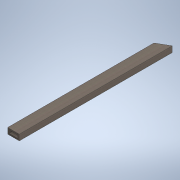
# Autodesk Inventor part: 1x0_5x12-aluminumExtrusion
Saved by Autodesk Inventor 2020.2 (Build 242310000, 310)
## iProperties
Created: 2020-01-20
Part Number: 1x0_5x12-aluminumExtrusion
Material: Aluminum 6061, Welded
Document SubType Name: Modeling
Designer: robst
Density: 2.7 g/cm^3
Appearance: Walnut
Author: robst
Autodesk Inventor part; units mm, degrees
ref_plane "YZ Plane" through (0, 0, 0) normal (1, 0, 0) x (0, 1, 0)
ref_plane "XZ Plane" through (0, 0, 0) normal (0, 1, 0) x (-1, 0, 0)
ref_plane "XY Plane" through (0, 0, 0) normal (0, 0, 1) x (1, 0, 0)
sketch "Sketch1" plane through (0, 0, 0) normal (0, 0, 1) x (1, 0, 0)
  line L0 (-12.7, -6.35) -> (12.7, -6.35)
  line L1 (12.7, -6.35) -> (12.7, 6.35)
  line L2 (12.7, 6.35) -> (-12.7, 6.35)
  line L3 (-12.7, 6.35) -> (-12.7, -6.35)
  line L4 (-12.7, -6.35) -> (12.7, 6.35) construction
  line L5 (12.7, -6.35) -> (-12.7, 6.35) construction
  line L6 (-9.525, -3.175) -> (9.525, -3.175)
  line L7 (9.525, -3.175) -> (9.525, 3.175)
  line L8 (9.525, 3.175) -> (-9.525, 3.175)
  line L9 (-9.525, 3.175) -> (-9.525, -3.175)
  line L10 (-9.525, -3.175) -> (9.525, 3.175) construction
  line L11 (9.525, -3.175) -> (-9.525, 3.175) construction
  point P0 (0, 0)
  dimension "d0" = 25.4
  dimension "d1" = 12.7
  dimension "d2" = 3.175
  dimension "d3" = 3.175
  constraints: 24 end point, 4 midpoint, 4 parallel, 2 horizontal, 2 perpendicular
  measures "d0" distance of L0.start L0.end
  measures "d1" distance of L1.end L0.end
  measures "d2" distance between parallel lines of L0 L6
  measures "d3" distance between parallel lines of L3 L9
extrude "Extrusion1" add sketch "Sketch1" along normal mid plane 334.137
sketch "Sketch2" plane through (-12.7, -6.35, 167.0685) normal (0, -1, 0) x (1, 0, 0)
  line L0 (25.4, -334.137) -> (0, -334.137) projected
  line L1 (25.4, -334.137) -> (0, -319.4723)
  line L2 (0, 0) -> (0, -334.137) projected
  line L3 (0, -334.137) -> (0, -319.4723)
  line L4 (0, -334.137) -> (25.4, -334.137)
  line L5 (22.225, -334.137) -> (22.225, 0) projected
  point P0 (12.7, -167.0685)
  dimension "d6" = 30
  constraints: 6 end point, 1 perpendicular, 1 point on line, 1 vertical
  measures "d6" angle of L0 L1
extrude "Extrusion2" cut sketch "Sketch2" against normal through all
body "Solid1"
